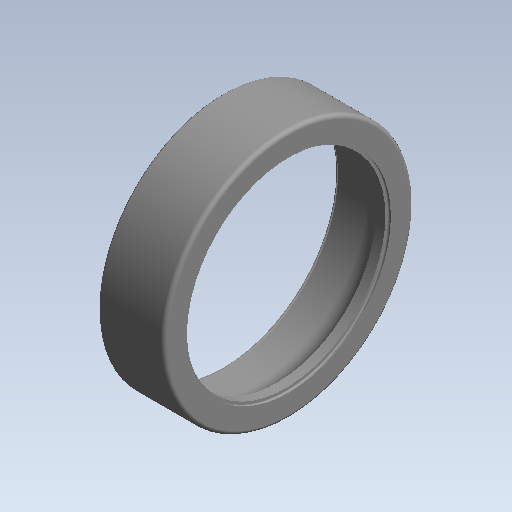
# Autodesk Inventor part: 7306 BE-2RZP_PART2
Saved by Autodesk Inventor 2020 (Build 240168000, 168)
## iProperties
Part Number: 7306 BE-2RZP_PART2
Material: Generic
Catalog Web Link: www.cadenas.de
Description: -Angular contact ball bearings, single row
Vendor: SKF
Document SubType Name: Modeling
Designer: partserver
Manufacturer: SKF
Mass: 18.5382 g
Surface Area: 105.726 cm^2
Volume: 18.5382 cm^3
Density: 1 g/cm^3
Appearance: PSOLRGB-175-175-175
Category: PARTsolutions
Company: SKF
PSOL_IDENT_0: {$CADENAS_DATA\23d-libs\skf\bearings_units_and_housings\ball_bearings\angular_contact_ball_bearings\
PSOL_IDENT_1: ba1_001_101.prj},204 {VTYP=3D},{NB=7306 BE-2RZP_PART2},{LINA=7306 BE-2RZP_PART2},{NN=BA1_001_101_PAR
PSOL_IDENT_2: T2},{NOPRJ=TRUE},{DATE=10.08.2020 12:45:11},{GEOMDATE=10.08.2020 08:19:26},{VERSION=},{LINEID=142100
PSOL_IDENT_3: },{WBVAR=},{WBNUMERIC=}  {NB=7306 BE-2RZP_PART2},{LINA=7306 BE-2RZP_PART2},{KT=DUMMY},{DESIGNATION=7
PSOL_IDENT_4: 306 BE-2RZP},{DD=30.000},{D=72.000},{B=19.0000},{DD1=46.500},{DD2=37.900},{D1=MIN},{D2=58.750},{D3=M
PSOL_IDENT_5: IN},{D4=64.260},{D5=64.85},{C1=MIN},{AA=31},{R12=1.100},{R34=0.600},{ALPHA=40},{PITCH=51.000},{DW=13
PSOL_IDENT_6: .494},{DDAMIN=37},{DDAMAX=46},{DAMAX=65},{DBMAX=67.8},{RAMAX=1},{RBMAX=0.6},{LOAD1=32.5},{LOAD2=19.3
PSOL_IDENT_7: },{LOAD3=0.815},{SPEED1=12000},{SPEED2=9500},{Z=10},{II=1},{MASS=0.35},{BEARING=7306 BE-2RZP},{POPUL
PSOL_IDENT_8: AR=Yes},{VARIANT=design_ba1_001_101_1},{D2A=58.75},{DD2A=37.900},{R5R=0.6},{R34L=1.1},{IRH=1},{ORH=1
PSOL_IDENT_9: },{D4H=1.1}
NB: 7306 BE-2RZP_PART2
NT: Angular contact ball bearings, single row
NBSYN: $DESIGNATION._PART2
LINA: 7306 BE-2RZP_PART2
CATALOG: SKF
SUPPLIER: SKF
ARTICLENO: 7306 BE-2RZP_PART2
BOMINFO: 7306 BE-2RZP_PART2
CREATOR: CADENAS GmbH
Title: 7306 BE-2RZP_PART2
Author: Cadenas PARTsolutions
Comments: Angular contact ball bearings, single row
Autodesk Inventor part; units mm, degrees
ref_plane "YZ Plane" through (0, 0, 0) normal (1, 0, 0) x (0, 1, 0)
ref_plane "XZ Plane" through (0, 0, 0) normal (0, 1, 0) x (-1, 0, 0)
ref_plane "XY Plane" through (0, 0, 0) normal (0, 0, 1) x (1, 0, 0)
sketch "Sketch_4" plane through (0, 0, 0) normal (0, 0, 1) x (1, 0, 0)
  line L0 (19, 0) -> (0, 0)
  line L1 (0, 34.9) -> (0, 29.375)
  line L2 (0, 29.375) -> (0.1833, 29.375)
  arc A0 (0.9167, 29.375) -> (0.1833, 29.375) centre (0.55, 29.375) ccw
  line L3 (0.9167, 29.375) -> (0.9167, 28.7125)
  line L4 (0.9167, 28.7125) -> (3.5669, 28.7125)
  arc A1 (9.5, 32.247) -> (3.5669, 28.7125) centre (9.5, 25.5) ccw
  line L5 (9.5, 32.247) -> (18.0833, 32.247)
  line L6 (18.0833, 32.247) -> (18.0833, 32.6875)
  arc A2 (18.8167, 32.6875) -> (18.0833, 32.6875) centre (18.45, 32.6875) ccw
  line L7 (18.8167, 32.6875) -> (19, 32.6875)
  line L8 (19, 32.6875) -> (19, 35.4)
  arc A3 (19, 35.4) -> (18.4, 36) centre (18.4, 35.4) ccw
  line L9 (18.4, 36) -> (1.1, 36)
  arc A4 (1.1, 36) -> (0, 34.9) centre (1.1, 34.9) ccw
  constraints: 20 end point, 10 point on circle, 5 centre point
revolve "Revolution1" add sketch "Sketch_4" angle 360 about axis through (19, 0, 0) along (1, 0, 0)
body "Solid1"
